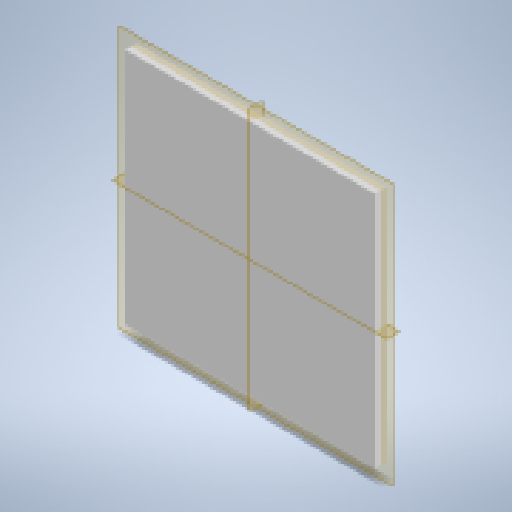
# Autodesk Inventor part: Крыло(подвижная часть)
Saved by Autodesk Inventor 2023.2 (Build 272271030, 271C)
## iProperties
Created: 2024-03-20
Part Number: Крыло(подвижная часть)
Material: Типовые
Document SubType Name: Modeling
Designer: I9232
Density: 1 g/cm^3
Appearance: По умолчанию
Author: I9232
Autodesk Inventor part; units mm, degrees
sketch "Эскиз1" plane through (0, 0, 0) normal (0, 0, 1) x (1, 0, 0)
  line L0 (-43.5, -41.5) -> (43.5, -41.5)
  line L1 (43.5, -41.5) -> (43.5, 41.5)
  line L2 (43.5, 41.5) -> (-43.5, 41.5)
  line L3 (-43.5, 41.5) -> (-43.5, -41.5)
  line L4 (-43.5, -41.5) -> (43.5, 41.5) construction
  line L5 (43.5, -41.5) -> (-43.5, 41.5) construction
  point P0 (0, 0)
  dimension "d0" = 87
  dimension "d1" = 83
  constraints: 12 end point, 2 midpoint, 2 parallel, 1 horizontal, 1 perpendicular
  measures "d0" distance of L1.end L2.end
  measures "d1" distance of L0.end L1.end
extrude "Выдавливание1" add sketch "Эскиз1" along normal mid plane 4
